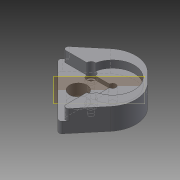
# Autodesk Inventor part: leveling clip
Saved by Autodesk Inventor 2014 (Build 180170000, 170)
## iProperties
Created: 2016-05-11
Part Number: leveling clip
Material: Generic
Document SubType Name: Modeling
Designer: eric.parent
Density: 1 g/cm^3
Appearance: Default
Author: eric.parent
Autodesk Inventor part; units mm, degrees
ref_plane "YZ Plane" through (0, 0, 0) normal (1, 0, 0) x (0, 1, 0)
ref_plane "XZ Plane" through (0, 0, 0) normal (0, 1, 0) x (-1, 0, 0)
ref_plane "XY Plane" through (0, 0, 0) normal (0, 0, 1) x (1, 0, 0)
sketch "Sketch1" plane through (0, 0, 0) normal (0, 0, 1) x (1, 0, 0)
  line L0 (102, 102) -> (102, 0) construction
  line L1 (0, 102) -> (102, 102) construction
  arc A0 (110.8376, 117.4467) -> (83.8397, 118.6255) centre (96.6954, 103.3046) ccw projected
  arc A1 (118.6255, 83.8397) -> (117.4467, 110.8376) centre (103.3046, 96.6954) ccw projected
  line L2 (110.8376, 117.4467) -> (117.4467, 110.8376)
  line L3 (83.8397, 118.6255) -> (64.0262, 102)
  line L4 (102, 64.0262) -> (118.6255, 83.8397)
  line L5 (64.0262, 102) -> (102, 64.0262)
  point P0 (0, 0)
  constraints: 8 end point, 3 tangent, 2 point on line, 1 parallel
extrude "Extrusion3" add sketch "Sketch1" along normal blind 15
sketch "Sketch3" plane through (0, 0, 15) normal (0, 0, 1) x (1, 0, 0)
  line L0 (64.0262, 102) -> (102, 102)
  line L1 (102, 102) -> (102, 64.0262)
  line L2 (64.0262, 102) -> (102, 64.0262)
  point P0 (0, 0)
  constraints: 6 end point, 1 horizontal, 1 perpendicular
extrude "Extrusion4" cut sketch "Sketch3" against normal blind 7.5
sketch "Sketch5" plane through (0, 0, 15) normal (0, 0, 1) x (1, 0, 0)
  line L0 (117.4467, 110.8376) -> (110.8376, 117.4467) construction
  line L1 (114.1421, 114.1421) -> (34.2284, 34.2284) construction
  line L2 (102, 64.0262) -> (64.0262, 102) construction
  circle A0 centre (90.0842, 90.0842) radius 6
  point P0 (0, 0)
  dimension "d25" = 12
  dimension "d26" = 10
  constraints: 2 end point, 1 centre point, 1 midpoint, 1 perpendicular, 1 point on line
  measures "d25" diameter of A0
  measures "d26" distance from line of L2 A0.centre
extrude "Extrusion6" cut sketch "Sketch5" against normal through all
sketch "Sketch6" plane through (0, 0, 15) normal (0, 0, 1) x (1, 0, 0)
  circle A0 centre (102, 102) radius 2.2
  point P0 (0, 0)
  dimension "d27" = 4.4
  constraints: 1 centre point, 1 coincident
  measures "d27" diameter of A0
extrude "Extrusion7" cut sketch "Sketch6" against normal through all
sketch "Sketch7" plane through (0, 0, 15) normal (0, 0, 1) x (1, 0, 0)
  arc A0 (102, 99.8) -> (99.8, 102) centre (102, 102) ccw construction
  circle A1 centre (102, 102) radius 15
  point P0 (0, 0)
  dimension "d30" = 30
  constraints: 1 centre point, 1 coincident
  measures "d30" diameter of A1
extrude "Extrusion8" cut sketch "Sketch7" against normal blind 5
sketch "Sketch8" plane through (0, 0, 15) normal (0, 0, 1) x (1, 0, 0)
  circle A0 centre (90.0842, 90.0842) radius 6 construction
  line L0 (102, 64.0262) -> (64.0262, 102) construction
  line L1 (62.2356, 117.9328) -> (118.3829, 61.7854) construction
  circle A1 centre (102, 87) radius 1.65
  point P0 (0, 0)
  dimension "d42" = 3.3
  constraints: 2 end point, 1 centre point, 1 coincident, 1 parallel, 1 point on line
  measures "d42" diameter of A1
extrude "Extrusion9" cut sketch "Sketch8" against normal through all
sketch "Sketch9" plane through (0, 0, 15) normal (0, 0, 1) x (1, 0, 0)
  arc A0 (102, 85.35) -> (103.6475, 87.0907) centre (102, 87) ccw projected
  circle A1 centre (102, 87) radius 3
  point P0 (0, 0)
  dimension "d43" = 6
  constraints: 1 centre point, 1 coincident
  measures "d43" diameter of A1
extrude "Extrusion10" cut sketch "Sketch9" against normal blind 10
ref_plane "Work Plane1" through (83.0131, 83.0131, 7.5) normal (0.7071068, -0.7071068, 0) x (0, 0, -1)
mirror "Mirror1" about plane through (83.0131, 83.0131, 7.5) normal (0.7071068, -0.7071068, 0) of "Extrusion9", "Extrusion10"
fillet "Fillet6" radius 2 4 edges at (64.0262, 102, 11.25) (64.0262, 102, 3.75) (102, 64.0262, 11.25) (102, 64.0262, 3.75)
body "Solid2"
